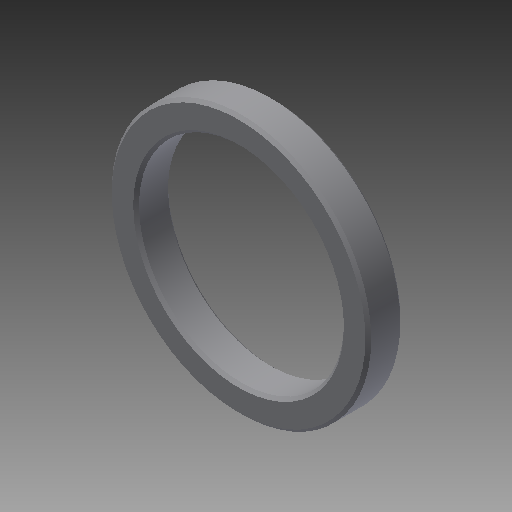
# Autodesk Inventor part: KE-SP-01
Saved by Autodesk Inventor 2018 (Build 220112000, 112)
## iProperties
Created: 2015-08-04
Part Number: KE-SP-01
Material: 一般
Document SubType Name: Modeling
Designer: ERIC
Density: 1 g/cm^3
Appearance: 預設
Author: ERIC
Autodesk Inventor part; units mm, degrees
ref_plane "YZ Plane" through (0, 0, 0) normal (1, 0, 0) x (0, 1, 0)
ref_plane "XZ Plane" through (0, 0, 0) normal (0, 1, 0) x (-1, 0, 0)
ref_plane "XY Plane" through (0, 0, 0) normal (0, 0, 1) x (1, 0, 0)
sketch "草圖1" plane through (0, 0, 0) normal (0, 0, 1) x (1, 0, 0)
  circle A0 centre (0, 0) radius 17.65
  circle A1 centre (0, 0) radius 22.35
  dimension "d0" = 44.7
  dimension "d1" = 35.3
  constraints: 2 centre point, 2 coincident
  measures "d0" diameter of A1
  measures "d1" diameter of A0
extrude "擠出1" add sketch "草圖1" along normal blind 6
chamfer "倒角1" distance 0.5 angle 45 4 edges at (-17.65, 0, 6) (-17.65, 0, 0) (-22.35, 0, 6) (-22.35, 0, 0)
